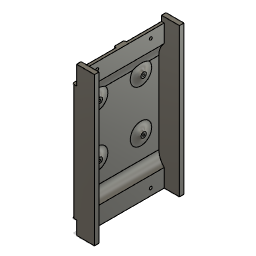
frame v7 (Autodesk Fusion 360 design; units mm, degrees)
Autodesk Fusion 360 part; units mm, degrees
sketch "スケッチ1" plane through (0, 0, 0) normal (0, 1, 0) x (1, 0, 0)
  line L0 (198.6513, 0) -> (-212.4639, 0) construction
  line L1 (0, -171.1167) -> (0, 175.9148) construction
  line L2 (0, 50) -> (0, -50)
  line L3 (-5, -50) -> (-5, 50)
  line L4 (-15, -50) -> (-15, 50)
  line L5 (-15, -50) -> (0, -50)
  line L6 (-15, 50) -> (0, 50)
  line L7 (-23.6283, -5) -> (8.2787, -5) construction
  line L8 (8.2787, 5) -> (-23.7559, 5) construction
  line L9 (-27.2019, -6) -> (16.7021, -6) construction
  line L10 (11.0865, 6) -> (-23.7559, 6) construction
  line L11 (-2.4, -5) -> (-2.4, 5)
  line L12 (-2.4, -5) -> (0, -6)
  line L13 (-2.4, 5) -> (0, 6)
  dimension "d3" = 5
  dimension "d4" = 50
  dimension "d5" = 100
  dimension "d6" = 15
  dimension "d28" = 5
  dimension "d29" = 1
  dimension "d30" = 10
  dimension "d31" = 12
  dimension "d32" = 2.4
  constraint horizontal L0
  constraint perpendicular L0 L1
  constraint vertical L2
  constraint coincident L1 L2.end
  constraint perpendicular L0 L4
  constraint perpendicular L1 L5
  constraint perpendicular L2 L6
  constraint perpendicular L2 L7
  constraint perpendicular L4 L8
  constraint perpendicular L3 L9
  constraint perpendicular L4 L10
  constraint coincident L7 L11.start
  constraint coincident L8 L11.end
  constraint perpendicular L8 L11
  constraint coincident L9 L12.end
  constraint coincident L1 L12.end
  constraint coincident L2 L13.end
  constraint coincident L10 L13.end
  measures "d3" distance of L2 L3
  measures "d4" distance of L0 L5
  measures "d5" distance of L5 L6
  measures "d6" distance of L1 L4
  measures "d28" distance of L0 L7
  measures "d29" distance of L7 L9
  measures "d30" distance of L7 L8
  measures "d31" distance of L9 L10
  measures "d32" distance of L2 L11
sketch "スケッチ2" plane through (0, 0, 0) normal (1, 0, 0) x (0, 0, -1)
  line L0 (100.9449, 0) -> (-99.6983, 0) construction
  line L1 (0, -52.919) -> (0, 192.9672) construction
  line L2 (50, 0) -> (-50, 0)
  line L3 (-50, 0) -> (-50, 160)
  line L4 (-50, 160) -> (50, 160)
  line L5 (50, 160) -> (50, 0)
  line L6 (-50, 0) -> (50, 0)
  line L7 (50, 145) -> (-50, 145)
  line L8 (50, 15) -> (-50, 15)
  line L9 (-45, 140) -> (45, 140)
  line L10 (45, 140) -> (45, 20)
  line L11 (45, 20) -> (-45, 20)
  line L12 (-45, 20) -> (-45, 140)
  line L13 (-71.2876, 152.5) -> (72.0089, 152.5) construction
  line L14 (-30, 173.4741) -> (-30, 123.8549) construction
  line L15 (-30, 123.8549) -> (-30, -28.7813) construction
  line L16 (30, 178.3367) -> (30, -29.5816) construction
  line L17 (-80.6344, 7.5) -> (85.0085, 7.5) construction
  line L18 (-171.1167, 0) -> (175.9148, 0) construction
  line L19 (45, 20) -> (45, 0)
  line L20 (-45, 20) -> (-45, 0)
  line L21 (45, 140) -> (45, 160)
  line L22 (-45, 140) -> (-45, 145)
  line L23 (-45, 160) -> (-45, 140)
  circle A0 centre (-30, 152.5) radius 1.6
  circle A1 centre (30, 152.5) radius 1.6
  circle A2 centre (-30, 7.5) radius 1.6
  circle A3 centre (30, 7.5) radius 1.6
  line L24 (-24, 118) -> (25, 118) construction
  line L25 (25, 118) -> (25, 60) construction
  line L26 (25, 60) -> (-24, 60) construction
  line L27 (-24, 60) -> (-24, 118) construction
  line L28 (22, 140) -> (22, 137.0697)
  circle A4 centre (-24, 118) radius 1.1
  circle A5 centre (25, 118) radius 1.1
  circle A6 centre (-24, 60) radius 1.1
  circle A7 centre (25, 60) radius 1.1
  circle A8 centre (-24, 118) radius 3
  circle A9 centre (25, 118) radius 3
  circle A10 centre (-24, 60) radius 3
  circle A11 centre (25, 60) radius 3
  dimension "d7" = 50
  dimension "d9" = 100
  dimension "d10" = 160
  dimension "d11" = 15
  dimension "d12" = 15
  dimension "d13" = 5
  dimension "d14" = 5
  dimension "d15" = 5
  dimension "d16" = 5
  dimension "d17" = 7.5
  dimension "d18" = 7.5
  dimension "d19" = 20
  dimension "d20" = 20
  dimension "d42" = 3.2
  dimension "d43" = 3.2
  dimension "d44" = 3.2
  dimension "d45" = 3.2
  dimension "d48" = 49
  dimension "d49" = 58
  dimension "d50" = 25
  dimension "d51" = 40
  dimension "d52" = 22
  dimension "d57" = 2.2
  dimension "d58" = 2.2
  dimension "d59" = 2.2
  dimension "d60" = 2.2
  dimension "d65" = 6
  dimension "d66" = 6
  dimension "d67" = 6
  dimension "d68" = 6
  constraint horizontal L0
  constraint perpendicular L0 L1
  constraint horizontal L2
  constraint vertical L3
  constraint horizontal L4
  constraint vertical L5
  constraint coincident L0 L2.start
  constraint coincident L5 L7.start
  constraint coincident L3 L7.end
  constraint perpendicular L3 L7
  constraint coincident L5 L8.start
  constraint coincident L3 L8.end
  constraint perpendicular L3 L8
  constraint horizontal L9
  constraint vertical L10
  constraint horizontal L11
  constraint vertical L12
  constraint perpendicular L5 L13
  constraint perpendicular L9 L14
  constraint perpendicular L2 L16
  constraint perpendicular L16 L17
  constraint perpendicular L6 L19
  constraint coincident L2 L19.end
  constraint perpendicular L0 L20
  constraint coincident L18 L20.end
  constraint perpendicular L7 L21
  constraint coincident L7 L22.end
  constraint perpendicular L7 L22
  constraint perpendicular L9 L23
  constraint coincident L4 L23.start
  constraint coincident L14 A0.centre
  constraint coincident L13 A0.centre
  constraint coincident L13 A1.centre
  constraint coincident L16 A1.centre
  constraint coincident L15 A2.centre
  constraint coincident L17 A2.centre
  constraint coincident L16 A3.centre
  constraint coincident L17 A3.centre
  constraint horizontal L24
  constraint vertical L25
  constraint horizontal L26
  constraint vertical L27
  constraint coincident L9 L28.start
  constraint perpendicular L9 L28
  constraint coincident L24.start L27.end
  constraint coincident L24.end L25.start
  constraint coincident L26.end L27.start
  constraint coincident L25.end L26.start
  constraint concentric A4 A8
  constraint concentric A5 A9
  constraint concentric A6 A10
  constraint concentric A7 A11
  measures "d7" distance of L1 L5
  measures "d9" distance of L3 L5
  measures "d10" distance of L4 L6
  measures "d11" distance of L6 L8
  measures "d12" distance of L4 L7
  measures "d13" distance of L3 L12
  measures "d14" distance of L5 L10
  measures "d15" distance of L7 L9
  measures "d16" distance of L8 L11
  measures "d17" distance of L4 L13
  measures "d18" distance of L17 L18
  measures "d19" distance of L3 L15
  measures "d20" distance of L5 L16
  measures "d42" diameter of A0
  measures "d43" diameter of A1
  measures "d44" diameter of A2
  measures "d45" diameter of A3
  measures "d48" distance of L25 L27
  measures "d49" distance of L24 L26
  measures "d50" distance of L1 L25
  measures "d51" distance of L11 L26
  measures "d52" distance of L9 L24
  measures "d57" diameter of A4
  measures "d58" diameter of A5
  measures "d59" diameter of A6
  measures "d60" diameter of A7
  measures "d65" diameter of A8
  measures "d66" diameter of A9
  measures "d67" diameter of A10
  measures "d68" diameter of A11
extrude "押し出し1" add sketch "スケッチ2" against normal blind 5 contours L5 L7 L8 L10 L19 L21 | L8 L11 L19 L20 | L3 L7 L8 L12 L20 L22 L23 | L7 L9 L21 L22 L23
extrude "押し出し2" add sketch "スケッチ2" along normal blind 2 from surface at -5 contours L9 L10 L11 L12 | A4 | A5 | A6 | A7 | A8 | A9 | A10 | A11
extrude "押し出し4" add sketch "スケッチ1" along normal up to surface (15 mm away) contours L2 L11 L12 L13
extrude "押し出し5" add 1 faces at (-0.8, 0, 1.6667) along direction (0, 1, 0) blind 15 from surface at 145
extrude "押し出し6" add sketch "スケッチ2" along normal blind 3 contours L2 L6 L8 L19 L20 | L8 L11 L19 L20 | L7 L9 L21 L22 L23 | L4 L7 L21 L23
extrude "押し出し7" add sketch "スケッチ2" along normal blind 20 contours L2 L5 L6 L8 L19 | L5 L7 L8 L10 L19 L21 | L2 L3 L6 L8 L20 | L4 L5 L7 L21 | L3 L7 L8 L12 L20 L22 L23 | L3 L4 L7 L23
fillet "フィレット1" radius 2 2 edges at (-5, 80, 50) (-5, 80, -50)
extrude "押し出し9" add sketch "スケッチ2" against normal up to surface (3 mm away) contours A8 | A9 | A10 | A11
sketch "スケッチ3" plane through (0, 160, 0) normal (0, 1, 0) x (-1, 0, 0)
  line L0 (2.4, -5) -> (2.4, 5)
  line L1 (2.4, 5) -> (0, 6)
  line L2 (0, 6) -> (0, 50)
  line L3 (0, 50) -> (-20, 50)
  line L4 (-20, 50) -> (-20, 45)
  line L5 (-20, 45) -> (-3, 45)
  line L6 (-3, 45) -> (-3, -45)
  line L7 (-3, -45) -> (-20, -45)
  line L8 (-20, -45) -> (-20, -50)
  line L9 (-20, -50) -> (0, -50)
  line L10 (0, -50) -> (0, -6)
  line L11 (0, -6) -> (2.4, -5)
  line L12 (-20, 50) -> (0, 50)
  line L13 (0, 50) -> (0, 45)
  line L14 (0, 45) -> (-20, 45)
  line L15 (-20, 45) -> (-20, 50)
  line L16 (-20, -50) -> (0, -50)
  line L17 (0, -50) -> (0, -45)
  line L18 (0, -45) -> (-20, -45)
  line L19 (-20, -45) -> (-20, -50)
  constraint horizontal L12
  constraint vertical L13
  constraint horizontal L14
  constraint vertical L15
  constraint coincident L2 L13.end
  constraint coincident L3.end L4.start
  constraint horizontal L16
  constraint vertical L17
  constraint horizontal L18
  constraint vertical L19
  constraint coincident L10 L17.end
  constraint coincident L8.end L9.start
extrude "押し出し10" add sketch "スケッチ3" along normal blind 6 contours L7 L8 L9 L10 L16 L17 L18 L19 | L2 L3 L4 L5 L12 L13 L14 L15
fillet "フィレット2" radius 20 1 edges at (-3, 140, 0)
fillet "フィレット3" radius 15 4 edges at (-3, 119.0848, 26.797) (-3, 119.0848, -22.203) (-3, 61.0848, 26.797) (-3, 61.0848, -22.203)
fillet "フィレット4" radius 20 1 edges at (-3, 20, 0)
